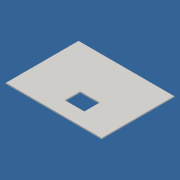
# Autodesk Inventor part: Cardboard_front
Saved by Autodesk Inventor 2016 (Build 200138000, 138)
## iProperties
Created: 2016-04-04
Part Number: Cardboard_front
Material: Generic
Document SubType Name: Modeling
Designer: admin
Density: 1 g/cm^3
Appearance: Default
Author: admin
Autodesk Inventor part; units mm, degrees
ref_plane "YZ Plane" through (0, 0, 0) normal (1, 0, 0) x (0, 1, 0)
ref_plane "XZ Plane" through (0, 0, 0) normal (0, 1, 0) x (-1, 0, 0)
ref_plane "XY Plane" through (0, 0, 0) normal (0, 0, 1) x (1, 0, 0)
sketch "Sketch1" plane through (0, 0, 0) normal (0, 0, 1) x (1, 0, 0)
  line L0 (-181.2286, 168.7686) -> (137.6222, 168.7686)
  line L1 (137.6222, 168.7686) -> (137.6222, -73.3492)
  line L2 (137.6222, -73.3492) -> (-181.2286, -73.3492)
  line L3 (-181.2286, -73.3492) -> (-181.2286, 168.7686)
  line L4 (-32.5, 25.5) -> (32.5, 25.5)
  line L5 (32.5, 25.5) -> (32.5, -25.5)
  line L6 (32.5, -25.5) -> (-32.5, -25.5)
  line L7 (-32.5, -25.5) -> (-32.5, 25.5)
  point P0 (0, 0)
  point P1 (0, 25.5)
  point P2 (32.5, 0)
  dimension "d0" = 65
  dimension "d1" = 51
  constraints: 16 end point, 4 parallel, 2 horizontal, 2 midpoint, 2 perpendicular, 1 horizontal alignment, 1 vertical alignment
  measures "d0" distance of L4.start L4.end
  measures "d1" distance of L6.end L4.start
extrude "Extrusion1" add sketch "Sketch1" along normal blind 3
body "Solid1"
